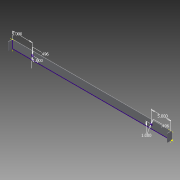
# Autodesk Inventor part: Bumpers
Saved by Autodesk Inventor 2015 (Build 190159000, 159)
## iProperties
Created: 2015-01-14
Part Number: Bumpers
Material: Generic
Document SubType Name: Modeling
Designer: chapale16
Density: 1 g/cm^3
Appearance: Default
Author: chapale16
Autodesk Inventor part; units mm, degrees
ref_plane "YZ Plane" through (0, 0, 0) normal (1, 0, 0) x (0, 1, 0)
ref_plane "XZ Plane" through (0, 0, 0) normal (0, 1, 0) x (-1, 0, 0)
ref_plane "XY Plane" through (0, 0, 0) normal (0, 0, 1) x (1, 0, 0)
sketch "Sketch1" plane through (0, 0, 0) normal (0, 0, 1) x (1, 0, 0)
  point P0 (0, 0)
sketch "Sketch2" plane through (0, 0, 0) normal (0, 0, 1) x (1, 0, 0)
  line L0 (0, 0) -> (-1022.35, 0)
  line L1 (-1022.35, 0) -> (-1022.35, 50.8)
  line L2 (-1022.35, 50.8) -> (0, 50.8)
  line L3 (0, 50.8) -> (0, 0)
  dimension "d0" = 50.8
  dimension "d1" = 1022.35
  constraints: 8 end point, 2 parallel, 1 horizontal, 1 perpendicular
  measures "d0" distance of L2.end L0.start
  measures "d1" distance of L0.start L0.end
extrude "Extrusion1" add sketch "Sketch2" along normal blind 3.175
sketch "Sketch3" plane through (0, 0, 3.175) normal (0, 0, 1) x (1, 0, 0)
  line L0 (0, 50.8) -> (-1022.35, 50.8) projected
  line L1 (0, 0) -> (-3.175, 0)
  line L2 (-3.175, 0) -> (-3.175, 50.8)
  line L3 (-3.175, 50.8) -> (0, 50.8)
  line L4 (0, 50.8) -> (0, 0)
  line L5 (-1022.35, 50.8) -> (-1019.175, 50.8)
  line L6 (-1019.175, 50.8) -> (-1019.175, 0)
  line L7 (-1019.175, 0) -> (-1022.35, 0)
  line L8 (-1022.35, 0) -> (-1022.35, 50.8)
  dimension "d4" = 3.175
  dimension "d5" = 3.175
  constraints: 16 end point, 4 parallel, 2 horizontal, 2 perpendicular, 1 point on line
  measures "d4" distance between parallel lines of L4 L2
  measures "d5" distance between parallel lines of L8 L6
extrude "Extrusion2" add sketch "Sketch3" along normal blind 25.4
sketch "Sketch4" plane through (0, 0, 3.175) normal (0, 0, 1) x (1, 0, 0)
  line L0 (-1019.175, 0) -> (-1019.175, 50.8)
  line L1 (-1019.175, 50.8) -> (-1019.175, 0) projected
  line L2 (-3.175, 0) -> (-3.175, 50.8)
  circle A0 centre (-892.175, 25.4) radius 6.2992
  circle A1 centre (-130.175, 25.4) radius 6.2992
  line L3 (-1019.175, 0) -> (-3.175, 0)
  line L4 (-1019.175, 0) -> (-3.175, 0) projected
  point P0 (0, 0)
  dimension "d8" = 12.5984
  dimension "d9" = 12.5984
  dimension "d10" = 25.4
  dimension "d11" = 127
  dimension "d12" = 127
  dimension "d13" = 25.4
  constraints: 6 end point, 2 centre point, 2 collinear, 1 vertical
  measures "d8" diameter of A0
  measures "d9" diameter of A1
  measures "d10" distance from line of L3 A1.centre
  measures "d11" distance from line of L2 A1.centre
  measures "d12" distance from line of L0 A0.centre
  measures "d13" distance from line of L3 A0.centre
body "Solid1"
